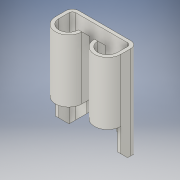
# Autodesk Inventor part: fuse clip
Saved by Autodesk Inventor 2019.3 (Build 233278000, 278)
## iProperties
Created: 2019-11-25
Part Number: fuse clip
Material: Generic
Document SubType Name: Modeling
Designer: kjdix
Density: 1 g/cm^3
Appearance: Steel
Author: kjdix
Autodesk Inventor part; units mm, degrees
ref_plane "YZ Plane" through (0, 0, 0) normal (1, 0, 0) x (0, 1, 0)
ref_plane "XY Plane" through (0, 0, 0) normal (0, 0, 1) x (1, 0, 0)
ref_plane "Work Plane1" through (0, 1.1938, 0) normal (0, 1, 0) x (-1, 0, 0)
sketch "Sketch1" plane through (0, 1.1938, 0) normal (0, 1, 0) x (-1, 0, 0)
  line L0 (0, 0) -> (0, -1.3462) construction
  line L1 (3.9624, -1.3462) -> (-3.9624, -1.3462)
  line L2 (4.9784, -0.3302) -> (4.9784, 1.2192)
  line L3 (-4.9784, -0.3302) -> (-4.9784, 1.2192)
  line L4 (4.9784, 3.2258) -> (0.9652, 3.2258) construction
  line L5 (0.9652, 3.2258) -> (0.9652, 1.2192) construction
  line L6 (-4.9784, 3.2258) -> (-0.9652, 3.2258) construction
  line L7 (-0.9652, 3.2258) -> (-0.9652, 1.2192) construction
  arc A0 (4.9784, 1.2192) -> (0.9652, 1.2192) centre (2.9718, 1.2192) ccw
  arc A1 (-0.9652, 1.2192) -> (-4.9784, 1.2192) centre (-2.9718, 1.2192) ccw
  line L8 (4.9784, 1.2192) -> (4.9784, 3.2258) construction
  line L9 (-4.9784, 1.2192) -> (-4.9784, 3.2258) construction
  arc A2 (3.9624, -1.3462) -> (4.9784, -0.3302) centre (3.9624, -0.3302) ccw
  arc A3 (-4.9784, -0.3302) -> (-3.9624, -1.3462) centre (-3.9624, -0.3302) ccw
  line L10 (0.9652, 1.2192) -> (0.9652, 0)
  line L11 (-0.9652, 1.2192) -> (-0.9652, 0)
  line L12 (-1.4732, 0) -> (-1.4732, 1.2192)
  arc A4 (-1.4732, 1.2192) -> (-4.4704, 1.2192) centre (-2.9718, 1.2192) ccw
  line L13 (-4.4704, 1.2192) -> (-4.4704, -0.3302)
  arc A5 (-4.4704, -0.3302) -> (-3.9624, -0.8382) centre (-3.9624, -0.3302) ccw
  line L14 (-3.9624, -0.8382) -> (3.9624, -0.8382)
  arc A6 (3.9624, -0.8382) -> (4.4704, -0.3302) centre (3.9624, -0.3302) ccw
  line L15 (4.4704, -0.3302) -> (4.4704, 1.2192)
  arc A7 (4.4704, 1.2192) -> (1.4732, 1.2192) centre (2.9718, 1.2192) ccw
  line L16 (1.4732, 1.2192) -> (1.4732, 0)
  line L17 (1.4732, 0) -> (0.9652, 0)
  line L18 (-0.9652, 0) -> (-1.4732, 0)
  line L19 (-4.9784, 1.2192) -> (-4.4704, 1.2192)
  line L20 (4.4704, 1.2192) -> (4.9784, 1.2192)
  point P0 (4.9784, -1.3462)
  point P1 (-4.9784, -1.3462)
  dimension "d1" = 1.3462
  dimension "d2" = 9.9568
  dimension "d3" = 4.572
  dimension "d4" = 4.572
  dimension "d5" = 1.9304
  dimension "d6" = 1.016
  dimension "d7" = 0.508
  constraints: 43 end point, 17 point on circle, 12 tangent, 8 centre point, 7 vertical, 5 horizontal, 5 point on line, 3 perpendicular, 2 collinear, 1 equal radius, 1 midpoint, 8 other
  measures "d1" distance of L0.end L0.start
  measures "d2" distance of point (4.978, -1.346) point (-4.978, -1.346)
  measures "d3" distance of point (4.978, -1.346) L4.start
  measures "d4" distance of point (-4.978, -1.346) L6.start
  measures "d5" distance between parallel lines of L7 L5
  measures "d6" radius of A2
  measures "d7" distance between parallel lines of L1 L14
extrude "Extrusion1" add sketch "Sketch1" along normal blind 9.525
extrude "Extrusion2" add sketch "Sketch1" against normal blind 5.1562 contours L1 A3 L3 L19 L13 A5 L14 A6 L15 L20 L2 A2
sketch "Sketch2" plane through (3.9624, 10.7188, -1.3462) normal (0, 0, -1) x (-1, 0, 0)
  line L0 (-0.508, 0) -> (-0.508, -14.6812) construction
  line L1 (-0.508, -14.6812) -> (-1.016, -14.1732)
  line L2 (-1.016, 0) -> (-1.016, -14.6812) construction
  line L3 (-0.508, -14.6812) -> (0.2104, -14.6812) construction
  line L4 (8.4328, 0) -> (8.4328, -14.6812) construction
  line L5 (8.4328, -14.6812) -> (8.9408, -14.1732)
  line L6 (8.9408, 0) -> (8.9408, -14.6812) construction
  line L7 (8.4328, -14.6812) -> (9.1512, -14.6812) construction
  line L8 (-0.508, -14.6812) -> (1.6764, -12.4968)
  line L9 (-0.508, -14.6812) -> (2.5812, -14.6812) construction
  line L10 (8.4328, -14.6812) -> (6.2484, -12.4968)
  line L11 (8.4328, -14.6812) -> (11.522, -14.6812) construction
  arc A0 (3.2004, -10.7188) -> (1.6764, -10.7188) centre (2.4384, -10.7188) ccw
  arc A1 (6.2484, -10.7188) -> (4.7244, -10.7188) centre (5.4864, -10.7188) ccw
  line L12 (1.6764, -12.4968) -> (1.6764, -10.7188)
  line L13 (6.2484, -12.4968) -> (6.2484, -10.7188)
  line L14 (4.7244, -10.7188) -> (3.2004, -10.7188)
  line L15 (-1.016, -14.1732) -> (-2.2198, -16.6808)
  line L16 (-2.2198, -16.6808) -> (9.9774, -16.6808)
  line L17 (9.9774, -16.6808) -> (8.9408, -14.1732)
  point P0 (3.9624, -10.7188)
  dimension "d12" = 135
  dimension "d13" = 45
  dimension "d14" = 45
  dimension "d15" = 135
  dimension "d16" = 4.572
  dimension "d17" = 1.524
  dimension "d18" = 1.524
  dimension "d19" = 0.762
  dimension "d20" = 0.762
  dimension "d21" = 0
  dimension "d22" = 0
  constraints: 28 end point, 5 equal length, 5 horizontal, 4 point on circle, 2 centre point, 2 point on line, 2 tangent, 1 perpendicular
  measures "d12" angle of L3 L1
  measures "d13" angle of L7 L5
  measures "d14" angle of L9 L8
  measures "d15" angle of L11 L10
  measures "d16" distance of L10.end L8.end
  measures "d17" diameter of A0
  measures "d18" diameter of A1
  measures "d19" horizontal distance of L8.end A0.centre
  measures "d20" horizontal distance of L10.end A1.centre
  measures "d21" vertical distance of point (3.962, -10.719) A0.centre
  measures "d22" vertical distance of point (3.962, -10.719) A1.centre
extrude "Extrusion3" cut sketch "Sketch2" against normal through all
sketch "Sketch3" plane through (4.9784, 10.7188, 1.2192) normal (1, 0, 0) x (0, 0, -1)
  line L0 (1.5494, -14.6812) -> (2.4293, -14.6812) projected
  line L1 (1.5494, -14.6812) -> (0, -13.1318)
  line L2 (0, -9.525) -> (0, -14.1732) projected
  line L3 (1.5494, -14.6812) -> (3.7406, -14.6812) construction
  line L4 (0, -13.1318) -> (-1.4703, -15.0958)
  line L5 (1.5494, 0) -> (1.5494, -14.6812) projected
  line L6 (-1.4703, -15.0958) -> (1.5494, -14.6812)
  point P0 (1.2192, -10.7188)
  dimension "d25" = 135
  constraints: 8 end point, 1 equal length, 1 horizontal, 1 point on line
  measures "d25" angle of L3 L1
extrude "Extrusion4" cut sketch "Sketch3" against normal through all
chamfer "Chamfer1" distance 1.2192 angle 45 2 edges at (-1.2192, 10.7188, 0) (1.2192, 10.7188, 0)
body "Solid1"
